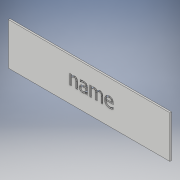
# Autodesk Inventor part: NamePlateV1
Saved by Autodesk Inventor 2019 (Build 230136000, 136)
## iProperties
Created: 2021-09-15
Part Number: NamePlateV1
Material: Generic
Document SubType Name: Modeling
Designer: timmy
Density: 1 g/cm^3
Appearance: Default
Author: timmy
Autodesk Inventor part; units mm, degrees
ref_plane "YZ Plane" through (0, 0, 0) normal (1, 0, 0) x (0, 1, 0)
ref_plane "XZ Plane" through (0, 0, 0) normal (0, 1, 0) x (-1, 0, 0)
ref_plane "XY Plane" through (0, 0, 0) normal (0, 0, 1) x (1, 0, 0)
sketch "Sketch1" plane through (0, 0, 0) normal (0, 0, 1) x (1, 0, 0)
  line L0 (0, 0) -> (609.6, 0)
  line L1 (609.6, 0) -> (609.6, 158.75)
  line L2 (609.6, 158.75) -> (0, 158.75)
  line L3 (0, 158.75) -> (0, 0)
  dimension "d0" = 609.6
  dimension "d1" = 158.75
  constraints: 8 end point, 2 parallel, 1 horizontal, 1 perpendicular
  measures "d0" distance of L2.end L1.end
  measures "d1" distance of L1.end L0.end
extrude "Extrusion1" add sketch "Sketch1" along normal blind 6.35
sketch "Sketch2" plane through (0, 0, 6.35) normal (0, 0, 1) x (1, 0, 0)
  line L0 (609.6, 158.75) -> (0, 158.75) projected
  line L1 (416.9921, 135.336) -> (416.9921, -23.414)
  line L2 (226.9609, 99.7712) -> (644.7194, 99.7712) construction
  line L3 (644.7194, 99.7712) -> (644.7194, 1.07) construction
  line L4 (644.7194, 1.07) -> (226.9609, 1.07) construction
  line L5 (226.9609, 1.07) -> (226.9609, 99.7712) construction
  line L6 (261.5411, 60.5803) -> (255.1191, 60.5803)
  line L7 (255.1191, 60.5803) -> (255.1191, 82.3164)
  spline S0 degree 2 poles (255.1191, 82.3164) (255.1191, 84.9511) (254.6251, 89.4795) (253.8841, 90.838) knots 0 0 0 1 2 2 2
  spline S1 degree 2 poles (253.8841, 90.838) (253.1019, 92.2788) (250.3026, 93.6785) (247.9149, 93.6785) knots 0 0 0 1 2 2 2
  spline S2 degree 2 poles (247.9149, 93.6785) (245.5272, 93.6785) (240.4637, 91.1261) (238.0348, 89.0678) knots 0 0 0 1 2 2 2
  line L8 (238.0348, 89.0678) -> (238.0348, 60.5803)
  line L9 (238.0348, 60.5803) -> (231.6128, 60.5803)
  line L10 (231.6128, 60.5803) -> (231.6128, 98.7009)
  line L11 (231.6128, 98.7009) -> (238.0348, 98.7009)
  line L12 (238.0348, 98.7009) -> (238.0348, 94.4607)
  spline S3 degree 2 poles (238.0348, 94.4607) (240.9165, 97.0542) (246.4741, 99.7712) (249.6027, 99.7712) knots 0 0 0 1 2 2 2
  spline S4 degree 2 poles (249.6027, 99.7712) (255.2014, 99.7712) (261.5411, 92.3612) (261.5411, 85.3216) knots 0 0 0 1 2 2 2
  line L13 (261.5411, 85.3216) -> (261.5411, 60.5803)
  spline S5 degree 2 poles (291.7988, 64.6146) (291.0167, 64.0383) (288.382, 61.98) (287.147, 61.3624) knots 0 0 0 1 2 2 2
  spline S6 degree 2 poles (287.147, 61.3624) (285.4591, 60.4568) (282.2893, 59.5099) (279.4076, 59.5099) knots 0 0 0 1 2 2 2
  spline S7 degree 2 poles (279.4076, 59.5099) (277.0611, 59.5099) (272.8209, 61.2801) (271.2154, 62.8856) knots 0 0 0 1 2 2 2
  spline S8 degree 2 poles (271.2154, 62.8856) (269.6922, 64.45) (267.8397, 69.0607) (267.8397, 71.613) knots 0 0 0 1 2 2 2
  spline S9 degree 2 poles (267.8397, 71.613) (267.8397, 75.565) (271.1742, 81.1637) (274.7969, 82.7693) knots 0 0 0 1 2 2 2
  spline S10 degree 2 poles (274.7969, 82.7693) (278.0079, 84.2513) (286.7353, 85.3628) (291.7988, 85.6509) knots 0 0 0 1 2 2 2
  line L14 (291.7988, 85.6509) -> (291.7988, 86.8859)
  spline S11 degree 2 poles (291.7988, 86.8859) (291.7988, 89.109) (290.4403, 91.8671) (289.2053, 92.6493) knots 0 0 0 1 2 2 2
  spline S12 degree 2 poles (289.2053, 92.6493) (287.9703, 93.4315) (284.43, 93.9255) (282.5363, 93.9255) knots 0 0 0 1 2 2 2
  spline S13 degree 2 poles (282.5363, 93.9255) (280.3133, 93.9255) (274.3029, 92.6082) (271.2977, 91.332) knots 0 0 0 1 2 2 2
  line L15 (271.2977, 91.332) -> (270.9272, 91.332)
  line L16 (270.9272, 91.332) -> (270.9272, 97.8775)
  spline S14 degree 2 poles (270.9272, 97.8775) (272.6974, 98.3715) (279.3253, 99.6065) (282.5775, 99.6065) knots 0 0 0 1 2 2 2
  spline S15 degree 2 poles (282.5775, 99.6065) (286.5295, 99.6065) (291.9223, 98.3715) (294.063, 96.766) knots 0 0 0 1 2 2 2
  spline S16 degree 2 poles (294.063, 96.766) (296.1625, 95.2017) (298.2209, 90.2205) (298.2209, 86.6389) knots 0 0 0 1 2 2 2
  line L17 (298.2209, 86.6389) -> (298.2209, 60.5803)
  line L18 (298.2209, 60.5803) -> (291.7988, 60.5803)
  line L19 (291.7988, 60.5803) -> (291.7988, 64.6146)
  line L20 (291.7988, 69.9663) -> (291.7988, 80.5462)
  spline S17 degree 2 poles (291.7988, 80.5462) (289.4935, 80.3404) (282.5363, 79.6406) (280.3544, 78.9819) knots 0 0 0 1 2 2 2
  spline S18 degree 2 poles (280.3544, 78.9819) (277.8021, 78.1997) (274.4676, 74.9475) (274.4676, 72.0659) knots 0 0 0 1 2 2 2
  spline S19 degree 2 poles (274.4676, 72.0659) (274.4676, 68.7725) (278.1726, 65.438) (281.7129, 65.438) knots 0 0 0 1 2 2 2
  spline S20 degree 2 poles (281.7129, 65.438) (284.7181, 65.438) (289.6582, 68.0315) (291.7988, 69.9663) knots 0 0 0 1 2 2 2
  line L21 (350.4617, 60.5803) -> (350.4617, 82.6458)
  spline S21 degree 2 poles (350.4617, 82.6458) (350.4617, 85.2804) (350.0501, 89.7676) (349.3914, 91.0026) knots 0 0 0 1 2 2 2
  spline S22 degree 2 poles (349.3914, 91.0026) (348.7327, 92.3612) (346.2215, 93.6785) (344.0397, 93.6785) knots 0 0 0 1 2 2 2
  spline S23 degree 2 poles (344.0397, 93.6785) (342.0637, 93.6785) (337.5353, 91.2496) (335.1476, 88.9443) knots 0 0 0 1 2 2 2
  spline S24 degree 2 poles (335.1476, 88.9443) (335.1888, 88.368) (335.2711, 86.7624) (335.2711, 85.6921) knots 0 0 0 1 2 2 2
  line L22 (335.2711, 85.6921) -> (335.2711, 60.5803)
  line L23 (335.2711, 60.5803) -> (328.8491, 60.5803)
  line L24 (328.8491, 60.5803) -> (328.8491, 82.6458)
  spline S25 degree 2 poles (328.8491, 82.6458) (328.8491, 85.2804) (328.4374, 89.7676) (327.7787, 91.0026) knots 0 0 0 1 2 2 2
  spline S26 degree 2 poles (327.7787, 91.0026) (327.1201, 92.3612) (324.6089, 93.6785) (322.427, 93.6785) knots 0 0 0 1 2 2 2
  spline S27 degree 2 poles (322.427, 93.6785) (320.3687, 93.6785) (315.7992, 91.085) (313.6585, 89.0678) knots 0 0 0 1 2 2 2
  line L25 (313.6585, 89.0678) -> (313.6585, 60.5803)
  line L26 (313.6585, 60.5803) -> (307.2364, 60.5803)
  line L27 (307.2364, 60.5803) -> (307.2364, 98.7009)
  line L28 (307.2364, 98.7009) -> (313.6585, 98.7009)
  line L29 (313.6585, 98.7009) -> (313.6585, 94.5018)
  spline S28 degree 2 poles (313.6585, 94.5018) (316.1697, 97.013) (321.1097, 99.7712) (324.0737, 99.7712) knots 0 0 0 1 2 2 2
  spline S29 degree 2 poles (324.0737, 99.7712) (327.4494, 99.7712) (332.6776, 96.6837) (334.0361, 93.1845) knots 0 0 0 1 2 2 2
  spline S30 degree 2 poles (334.0361, 93.1845) (336.959, 96.4367) (342.4753, 99.7712) (345.6864, 99.7712) knots 0 0 0 1 2 2 2
  spline S31 degree 2 poles (345.6864, 99.7712) (348.1564, 99.7712) (352.1907, 98.248) (353.6728, 96.519) knots 0 0 0 1 2 2 2
  spline S32 degree 2 poles (353.6728, 96.519) (355.1959, 94.79) (356.8838, 89.603) (356.8838, 85.6921) knots 0 0 0 1 2 2 2
  line L30 (356.8838, 85.6921) -> (356.8838, 60.5803)
  line L31 (356.8838, 60.5803) -> (350.4617, 60.5803)
  spline S33 degree 2 poles (382.4484, 59.7158) (373.3094, 59.7158) (363.2646, 69.9663) (363.2646, 79.4347) knots 0 0 0 1 2 2 2
  spline S34 degree 2 poles (363.2646, 79.4347) (363.2646, 88.7385) (373.0212, 99.7712) (380.8841, 99.7712) knots 0 0 0 1 2 2 2
  spline S35 degree 2 poles (380.8841, 99.7712) (384.4245, 99.7712) (389.8997, 97.7129) (391.9168, 95.531) knots 0 0 0 1 2 2 2
  spline S36 degree 2 poles (391.9168, 95.531) (393.9752, 93.3492) (396.157, 87.0506) (396.157, 82.4811) knots 0 0 0 1 2 2 2
  line L32 (396.157, 82.4811) -> (396.157, 78.9819)
  line L33 (396.157, 78.9819) -> (369.769, 78.9819)
  spline S37 degree 2 poles (369.769, 78.9819) (369.769, 72.354) (376.4381, 65.3145) (382.3661, 65.3145) knots 0 0 0 1 2 2 2
  spline S38 degree 2 poles (382.3661, 65.3145) (384.4656, 65.3145) (388.5411, 66.2613) (390.1878, 67.0023) knots 0 0 0 1 2 2 2
  spline S39 degree 2 poles (390.1878, 67.0023) (391.9168, 67.8257) (394.3045, 69.2665) (395.0867, 69.9252) knots 0 0 0 1 2 2 2
  line L34 (395.0867, 69.9252) -> (395.4572, 69.9252)
  line L35 (395.4572, 69.9252) -> (395.4572, 62.9268)
  spline S40 degree 2 poles (395.4572, 62.9268) (394.3457, 62.474) (390.97, 61.1566) (389.6527, 60.7861) knots 0 0 0 1 2 2 2
  spline S41 degree 2 poles (389.6527, 60.7861) (387.8001, 60.2509) (384.7538, 59.7158) (382.4484, 59.7158) knots 0 0 0 1 2 2 2
  spline S42 degree 2 poles (389.8997, 83.8808) (389.8173, 86.4743) (388.747, 90.2616) (387.7178, 91.5378) knots 0 0 0 1 2 2 2
  spline S43 degree 2 poles (387.7178, 91.5378) (386.6063, 92.9787) (383.1071, 94.5018) (380.5136, 94.5018) knots 0 0 0 1 2 2 2
  spline S44 degree 2 poles (380.5136, 94.5018) (377.9612, 94.5018) (374.3797, 92.9787) (372.8977, 91.4966) knots 0 0 0 1 2 2 2
  spline S45 degree 2 poles (372.8977, 91.4966) (371.4569, 89.9735) (369.9749, 86.3096) (369.769, 83.8808) knots 0 0 0 1 2 2 2
  line L36 (369.769, 83.8808) -> (389.8997, 83.8808)
  point P0 (0, 0)
  point P1 (304.8, 79.375)
  constraints: 2 end point, 1 vertical, 2 other
extrude "Extrusion2" cut sketch "Sketch2" against normal blind 6.35
body "Solid1"
